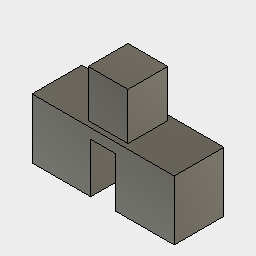
Switch Block (Autodesk Fusion 360 design; units mm, degrees)
Autodesk Fusion 360 part; units mm, degrees
box "BoxPrimitive1" add length 3.5 width 10 height 7 placed x (0, 1, 0) y (-1, 0, 0) z (0, 0, 1) at (10, 0, 0)
sketch "Sketch2" plane through (0, 0, 7) normal (0, 0, 1) x (-1, 0, 0)
  line L0 (-10, -3.5) -> (0, -3.5)
  line L1 (0, -3.5) -> (0, 0)
  line L2 (0, 0) -> (-10, 0)
  line L3 (-10, 0) -> (-10, -3.5)
  line L4 (-5, -3.5) -> (-5, -1.75)
  line L5 (-6.4, -0.35) -> (-3.6, -0.35)
  line L6 (-3.6, -0.35) -> (-3.6, -3.15)
  line L7 (-3.6, -3.15) -> (-6.4, -3.15)
  line L8 (-6.4, -3.15) -> (-6.4, -0.35)
  line L9 (-6.4, -0.35) -> (-3.6, -3.15) construction
  line L10 (-3.6, -0.35) -> (-6.4, -3.15) construction
  point P0 (-5, -1.75)
  dimension "d6" = 1.75
  dimension "d7" = 2.8
  dimension "d8" = 2.8
  measures "d6" distance of L4.start P0
  measures "d7" distance of L5.end L6.end
  measures "d8" distance of L6.end L7.end
extrude "Extrude1" cut sketch "Sketch2" against normal blind 3.5
sketch "Sketch3" plane through (0, 0, 0) normal (0, 0, -1) x (1, 0, 0)
  line L0 (0, -3.5) -> (10, -3.5)
  line L1 (10, -3.5) -> (10, 0)
  line L2 (10, 0) -> (0, 0)
  line L3 (0, 0) -> (0, -3.5)
  line L4 (5.875, -2.625) -> (4.125, -2.625)
  line L5 (4.125, -2.625) -> (4.125, -0.875)
  line L6 (4.125, -0.875) -> (5.875, -0.875)
  line L7 (5.875, -0.875) -> (5.875, -2.625)
  line L8 (5.875, -2.625) -> (4.125, -0.875) construction
  line L9 (4.125, -2.625) -> (5.875, -0.875) construction
  line L10 (4.125, -0.875) -> (5.875, -0.875)
  line L11 (5.875, -0.875) -> (5.875, 0)
  line L12 (5.875, 0) -> (4.125, 0)
  line L13 (4.125, 0) -> (4.125, -0.875)
  point P0 (5, -1.75)
  point P1 (5, -1.75)
  dimension "d11" = 1.75
  dimension "d12" = 1.75
  dimension "d17" = 1.75
  measures "d11" distance of L5.end L6.end
  measures "d12" distance of L4.end L5.end
  measures "d17" distance of L5.end L6.end
extrude "Extrude2" cut sketch "Sketch3" against normal blind 3.5 contours L4 L5 L6 L7 L10
extrude "Extrude3" add sketch "Sketch2" along normal blind 1 contours L5 L6 L7 L8
extrude "Extrude4" cut sketch "Sketch3" against normal blind 3.5 contours L2 L6 L10 L11 L12 L13
extrude "Extrude5" add 1 faces at (8.8, 1.2833, 3.5) along direction (0, 0, 1) blind 0.7
sketch "Sketch4" plane through (0, 0.35, 0) normal (0, -1, 0) x (1, 0, 0)
  line L0 (5.875, 4.2) -> (6.4, 4.2)
  line L1 (6.4, 4.2) -> (6.4, 8)
  line L2 (6.4, 8) -> (3.6, 8)
  line L3 (3.6, 8) -> (3.6, 4.2)
  line L4 (3.6, 4.2) -> (4.125, 4.2)
  line L5 (4.125, 4.2) -> (4.125, 3.5)
  line L6 (4.125, 3.5) -> (5.875, 3.5)
  line L7 (5.875, 3.5) -> (5.875, 4.2)
  line L8 (4.125, 3.5) -> (5.875, 3.5)
  line L9 (5.875, 3.5) -> (5.875, 4.2)
  line L10 (5.875, 4.2) -> (4.125, 4.2)
  line L11 (4.125, 4.2) -> (4.125, 3.5)
extrude "Extrude6" add sketch "Sketch4" along normal blind 0.35 contours L5 L6 L7 L8 L9 L10 L11
extrude "Extrude7" cut 1 faces at (5.4667, 1.2833, 8) along direction (0, 0, -1) blind 0.5
named bodies: "Switch Block"
